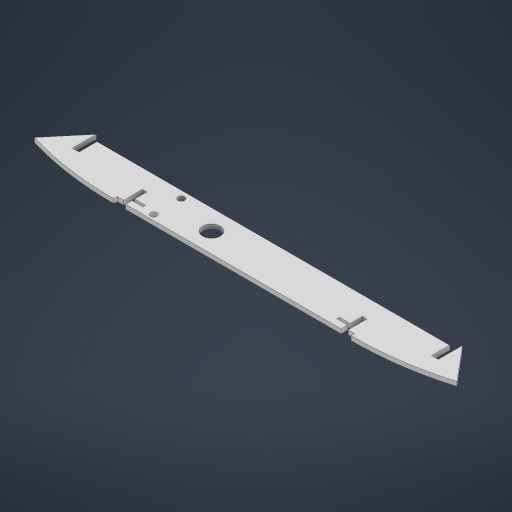
# Autodesk Inventor part: transom
Saved by Autodesk Inventor 2023 (Build 270158030, 158C)
## iProperties
Created: 2022-03-21
Part Number: transom
Material: Generic
Document SubType Name: Modeling
Designer: kardo
Density: 1 g/cm^3
Appearance: Default
Author: kardo
Autodesk Inventor part; units mm, degrees
ref_plane "YZ Plane" through (0, 0, 0) normal (1, 0, 0) x (0, 1, 0)
ref_plane "XZ Plane" through (0, 0, 0) normal (0, 1, 0) x (-1, 0, 0)
ref_plane "XY Plane" through (0, 0, 0) normal (0, 0, 1) x (1, 0, 0)
derived "parameters_frame.ipt"
derived "stencil_frame.ipt"
sketch "sk_joint_locations" plane through (81.12, 0, 0) normal (1, 0, 0) x (0, 1, 0)
  line L0 (0, 0) -> (111.39, 7.7891) construction
  line L1 (30.81, 28.832) -> (94.8, 28.832) construction
  arc A0 (30.81, 28.832) -> (9.48, 28.4869) centre (30.81, -630.4631) ccw construction
  line L2 (-254.1001, 19.9549) -> (9.48, 28.4869) construction
  line L3 (-363, 18.496) -> (-275.8801, 19.4795) construction
  arc A1 (-275.8801, 19.4795) -> (-254.1001, 19.9549) centre (-287.5515, 1053.3708) ccw construction
  line L4 (1.436, 1580.2049) -> (243.9436, -1887.8151) construction
  line L5 (-242.0001, 1541.8302) -> (-242.0001, -1877.3857) construction
  line L6 (-120.9999, 1541.8302) -> (-120.9999, -1877.3857) construction
  line L7 (-363, 1541.8302) -> (-363, -1877.3857) construction
  line L8 (0, 1541.8302) -> (0, -1877.3857) construction
  line L9 (445.406, 43.7257) -> (-613.1443, 6.7603) construction
  line L10 (-676.709, -27.4448) -> (497.0858, 54.635) construction
  line L11 (178.2183, 30.3929) -> (177.9391, 38.388) construction
  line L12 (185.9231, 36.8959) -> (186.4825, 28.8959) construction
  line L13 (0, 6.528) -> (111.1168, 11.6964) construction
  line L14 (-242.0001, 45.8501) -> (-242.0001, 20.3465) construction
  line L15 (-363, 37.4293) -> (-363, 18.496) construction
  line L16 (-120.9999, 51.0063) -> (-120.9999, 24.2633) construction
  line L17 (0, 52.89) -> (0, 28.18) construction
  line L18 (108.3896, 50.6971) -> (108.935, 42.897) construction
  line L19 (109.4805, 35.0968) -> (108.935, 42.897) construction
  line L20 (109.4805, 35.0968) -> (110.0259, 27.2967) construction
  line L21 (110.0259, 27.2967) -> (110.5713, 19.4965) construction
  line L22 (110.5713, 19.4965) -> (111.1168, 11.6964) construction
  line L23 (0, 6.528) -> (0, 0) construction
  spline S0 degree 4 poles (-363, 37.4293) (-272.3626, 45.1427) (-181.5879, 49.7528) (-90.8131, 52.89) (0, 52.89) knots 0 0 0 0 0 1 1 1 1 1
  spline S1 degree 3 poles (0, 52.89) (86.3106, 52.89) (181.3207, 49.5034) (237, 36.448) knots 0 0 0 0 1 1 1 1
  spline S2 degree 2 poles (111.39, 7.7891) (176.0348, 12.3096) (237, 36.448) knots 0 0 0 1 1 1
  line L24 (94.8, 37.536) -> (94.8, 28.832) construction
  line L25 (94.8, 35.548) -> (94.8, 30.82) construction
  point P0 (1.436, 1580.2049)
  point P1 (243.9436, -1887.8151)
  point P2 (178.0787, 34.3904)
  point P3 (186.2028, 32.8959)
  point P4 (134.9575, 11.3411)
  point P5 (-363, 27.9627)
  point P6 (-242.0001, 33.0983)
  point P7 (-120.9999, 37.6348)
  point P8 (0, 40.535)
  point P9 (94.8, 33.184)
sketch "sk_rudder_joint" plane through (0, -363, 0) normal (0, 1, 0) x (-1, 0, 0)
  line L0 (54.6, -1877.3857) -> (54.6, 1541.8302) construction
  line L1 (0, 18.496) -> (54.6, 18.496) construction
  line L2 (39, 35.696) -> (39, 22.996) construction
  line L3 (39, 29.346) -> (139, 29.346) construction
  line L4 (139, 29.346) -> (139, 129.346) construction
  line L5 (139, 129.346) -> (39, 129.346) construction
  line L6 (39, 129.346) -> (39, 35.696) construction
  point P0 (0, 0)
  point P1 (0, 39.712)
  point P2 (19, 24.846)
sketch3d "sk_servo_rod"
sketch "sk_cowl_joint_locations" plane through (54.6, 0, 0) normal (1, 0, 0) x (0, 1, 0)
  line L0 (-363, 18.496) -> (-275.8801, 19.4795) construction
  arc A0 (-275.8801, 19.4795) -> (-254.1001, 19.9549) centre (-287.5515, 1053.3708) ccw construction
  line L1 (-254.1001, 19.9549) -> (9.48, 28.4869) construction
  arc A1 (30.81, 28.832) -> (9.48, 28.4869) centre (30.81, -630.4631) ccw construction
  line L2 (30.81, 28.832) -> (94.8, 28.832) construction
  line L3 (94.8, 30.032) -> (30.81, 30.032) construction
  arc A2 (30.81, 30.032) -> (9.4412, 29.6862) centre (30.81, -630.4631) ccw construction
  line L4 (9.4412, 29.6862) -> (-254.1389, 21.1542) construction
  arc A3 (-275.8936, 20.6794) -> (-254.1389, 21.1542) centre (-287.5515, 1053.3708) ccw construction
  line L5 (-275.8936, 20.6794) -> (-363, 19.6961) construction
  line L6 (-242.0001, 1541.8302) -> (-242.0001, -1877.3857) construction
  line L7 (-120.9999, 1541.8302) -> (-120.9999, -1877.3857) construction
  line L8 (-363, 1541.8302) -> (-363, -1877.3857) construction
  line L9 (0, 1541.8302) -> (0, -1877.3857) construction
  line L10 (-242.0001, 45.0688) -> (-242.0001, 21.5472) construction
  line L11 (-120.9999, 49.9661) -> (-120.9999, 25.4639) construction
  line L12 (-363, 19.6961) -> (-363, 19.6961)
  line L13 (-363, 19.6961) -> (-363, 36.9211) construction
  line L14 (-513.5712, 1550.2518) -> (344.0815, -1889.6051) construction
  line L15 (-362.7741, 36.9211) -> (-363, 39.712) construction
  line L16 (0, 51.6) -> (0, 29.3806) construction
  spline S0 degree 2 poles (-363, 39.712) (-181.6483, 54.394) (0, 54.4) knots 0 0 0 1 1 1
  spline S1 degree 3 poles (0, 54.4) (31.284, 54.4) (68.256, 47.9917) (94.8, 37.536) knots 1 1 1 1 2 2 2 2
  spline S2 degree 3 poles (93.7738, 34.9308) (89.4268, 36.6431) (81.2968, 39.4556) (71.234, 42.2519) (63.4432, 44.1558) (58.1419, 45.3261) (51.4169, 46.6598) (45.9725, 47.6212) (39.1225, 48.6857) (33.6211, 49.4253) (26.7536, 50.2046) (21.2812, 50.7098) (14.5037, 51.1886) (7.8073, 51.5121) (2.5751, 51.6) (0, 51.6) knots 1 1 1 1 1.166667 1.291667 1.333333 1.416667 1.458333 1.541667 1.583333 1.666667 1.708333 1.791667 1.833333 1.916667 2 2 2 2
  spline S3 degree 3 poles (0, 51.6) (-20.1706, 51.5993) (-55.4643, 51.3605) (-95.7903, 50.6123) (-126.0307, 49.8474) (-146.1889, 49.2356) (-171.3841, 48.3435) (-191.5382, 47.528) (-216.7283, 46.3813) (-236.8783, 45.3621) (-262.0632, 43.9608) (-282.2091, 42.7379) (-307.3889, 41.082) (-332.5661, 39.2987) (-352.7052, 37.7363) (-362.7741, 36.9211) knots 0 0 0 0 0.166667 0.291667 0.333333 0.416667 0.458333 0.541667 0.583333 0.666666 0.708333 0.791666 0.833333 0.916666 1 1 1 1
  line L17 (-142.5135, 45.4866) -> (-137.389, 24.9334) construction
  line L18 (-134.789, 31.0394) -> (-138.6702, 30.0717) construction
  line L19 (-137.3512, 41.316) -> (-141.2324, 40.3483) construction
  line L20 (-142.5135, 45.4866) -> (-138.6324, 46.4543) construction
  line L21 (-137.389, 24.9334) -> (-133.5079, 25.9011) construction
  line L22 (-138.6324, 46.4543) -> (-138.8117, 52.2515) construction
  point P0 (0, 0)
  point P1 (-363, 28.3086)
  point P2 (-242.0001, 33.308)
  point P3 (-120.9999, 37.715)
  point P4 (0, 40.4903)
  point P5 (-513.5712, 1550.2518)
  point P6 (344.0815, -1889.6051)
  point P7 (-85.2629, 50.788)
  point P8 (0, 40.4903)
sketch "sk_transom_base" plane through (0, -363, 0) normal (0, 1, 0) x (-1, 0, 0)
  line L0 (-54.6, 39.712) -> (0, 39.712) construction
  spline S0 degree 2 poles (-54.6, 39.712) (-110.7355, 39.712) (-156, 0.6954) knots 0 0 0 1 1 1 construction
  line L1 (0, -967.2299) -> (0, 1390.1376) construction
  line L2 (-54.6, -967.2299) -> (-54.6, 1390.1376) construction
  line L3 (-81.12, -967.2299) -> (-81.12, 1390.1376) construction
  line L4 (-810.6605, 880.8565) -> (474.638, -650.9026) construction
  line L5 (-97.1551, 32.4008) -> (-84.12, 16.8661)
  line L6 (-84.12, 16.8661) -> (-84.12, 27.9627)
  line L7 (-84.12, 27.9627) -> (-81.12, 27.9627)
  line L8 (-81.12, 27.9627) -> (-81.12, 19.696)
  line L9 (-81.12, 19.696) -> (0, 19.696)
  line L10 (0, 38.112) -> (0, 19.696)
  line L11 (-54.6, 38.512) -> (-54.6, 38.112)
  line L12 (-54.6, 38.112) -> (0, 38.112)
  spline S1 degree 5 poles (-54.6, 38.512) (-65.4343, 38.5115) (-76.2676, 37.5985) (-87.0012, 35.6766) (-108.3164, 29.6774) (-128.1301, 19.7736) (-137.7, 13.8135) (-146.7224, 7.1082) (-155.2165, -0.2135) knots 0 0 0 0 0 0 0.491391 0.491391 0.491391 1 1 1 1 1 1
  point P0 (0, 0)
  point P1 (-34.32, 18.496)
  dimension "d3" = 1.2
  dimension "d2" = 1.2
  dimension "d4" = 3
  dimension "d5" = 1.2
  dimension "d36" = 1.6
  constraints: 16 end point, 3 perpendicular, 2 collinear, 2 parallel, 2 point on line, 4 other
  measures "d2" distance between parallel lines of L4 L5
  measures "d4" distance of L6.end L7.end
  measures "d5" distance from line of L9 point (-34.32, 18.496)
  measures "d36" distance between parallel lines of L0 L12
extrude "thicken" add sketch "sk_transom_base" along normal blind 2
sketch "sk_cut_joint" plane through (0, -363, 0) normal (0, 1, 0) x (-1, 0, 0)
  line L0 (-54.6, 39.712) -> (0, 39.712) projected
  line L1 (-54.6, -967.2299) -> (-54.6, 1390.1376) construction
  line L2 (-49.6, 39.712) -> (-49.6, 28.3086)
  line L3 (-49.6, 28.3086) -> (-51.6, 28.3086)
  line L4 (-51.6, 28.3086) -> (-51.6, 39.712)
  point P0 (0, 0)
  point P1 (-54.6, 28.3086)
  dimension "d25" = 2
  dimension "d26" = 5
  constraints: 6 end point, 3 parallel, 3 point on line
  measures "d25" distance between parallel lines of L2 L4
  measures "d26" distance between parallel lines of L2 L1
extrude "cut_joint" cut sketch "sk_cut_joint" along normal through all both and the other way through all
sketch "sk_cut_liner" plane through (0, -363, 0) normal (0, 1, 0) x (-1, 0, 0)
  line L0 (-54.6, 39.712) -> (0, 39.712) construction
  line L1 (-54.6, -967.2299) -> (-54.6, 1390.1376) projected
  line L2 (-44.6, 39.712) -> (-44.6, 33.912)
  line L3 (-44.6, 33.912) -> (-49.6, 33.912)
  line L4 (-49.6, 33.912) -> (-49.6, 36.912)
  line L5 (-49.6, 36.912) -> (-54.6, 36.912)
  line L6 (-44.6, 35.112) -> (-49.6, 35.112)
  line L7 (-49.6, 39.712) -> (-49.6, 36.912)
  line L8 (-49.6, 39.712) -> (-54.6, 39.712)
  point P0 (0, 0)
  dimension "d29" = 5
  dimension "d30" = 5
  dimension "d31" = 3
  dimension "d32" = 2.8
  dimension "d33" = 1.2
  constraints: 14 end point, 6 parallel, 5 point on line
  measures "d29" distance between parallel lines of L1 L4
  measures "d30" distance between parallel lines of L4 L2
  measures "d31" distance between parallel lines of L5 L3
  measures "d32" distance between parallel lines of L0 L5
  measures "d33" distance between parallel lines of L3 L6
extrude "cut_liner" cut sketch "sk_cut_liner" along normal through all both and the other way through all
mirror "mirror" about plane through (0, 0, 0) normal (1, 0, 0)
hole "drill_rudder" at (-39, -363, 35.696) at (-39, -363, 22.996) direction (0, 1, 0) diameter 3 end through all
hole "drill_servo_rod" at (-19.1351, -363, 29.0719) direction (0, 1, 0) diameter 8 end through all
equation "\"d3\" = shell_thickness"
equation "\"d2\" = shell_thickness"
equation "\"d4\" = stringer_thickness"
equation "\"d5\" = shell_thickness"
equation "\"d36\" = cowl_shell_thickness"
equation "\"d7\" = bulkhead_thickness"
equation "\"d25\" = bulkhead_thickness"
equation "\"d26\" = cowl_liner_width"
equation "\"d29\" = cowl_liner_width"
equation "\"d30\" = cowl_sealing_width"
equation "\"d31\" = cowl_sealing_thickness"
equation "\"d32\" = cowl_shell_thickness + cowl_liner_thickness"
equation "\"d33\" = cowl_liner_thickness"
equation "\"d9\" = drill_rudder_mount_diam"
equation "\"d18\" = drill_servo_rod_diam"
equation "\"shell_thickness\" = 1.2"
equation "\"stringer_thickness\" = 3"
equation "\"cowl_shell_thickness\" = 1.6"
equation "\"bulkhead_thickness\" = 2"
equation "\"cowl_liner_width\" = 5"
equation "\"cowl_sealing_width\" = 5"
equation "\"cowl_sealing_thickness\" = 3"
equation "\"cowl_liner_thickness\" = 1.2"
equation "\"drill_rudder_mount_diam\" = 3"
equation "\"drill_servo_rod_diam\" = 8"
body "Solid1"
